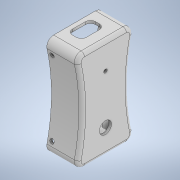
# Autodesk Inventor part: Bottom
Saved by Autodesk Inventor 2021 (Build 250183000, 183)
## iProperties
Created: 2024-02-01
Part Number: Bottom
Material: Generic
Document SubType Name: Modeling
Designer: maxsm
Density: 1 g/cm^3
Appearance: Default
Author: maxsm
Autodesk Inventor part; units mm, degrees
ref_plane "YZ Plane" through (0, 0, 0) normal (1, 0, 0) x (0, 1, 0)
ref_plane "XZ Plane" through (0, 0, 0) normal (0, 1, 0) x (-1, 0, 0)
ref_plane "XY Plane" through (0, 0, 0) normal (0, 0, 1) x (1, 0, 0)
sketch "Sketch1" plane through (0, 0, 0) normal (0, 1, 0) x (-1, 0, 0)
  line L0 (9, 13.5) -> (-9, 13.5)
  line L1 (-9, 13.5) -> (-9, -13.5)
  line L2 (-9, -13.5) -> (9, -13.5)
  line L3 (9, -13.5) -> (9, 13.5)
  line L4 (9, 13.5) -> (-9, -13.5) construction
  line L5 (-9, 13.5) -> (9, -13.5) construction
  point P0 (0, 0)
  dimension "d0" = 18
  dimension "d1" = 27
  constraints: 12 end point, 2 midpoint, 2 parallel, 1 horizontal, 1 perpendicular
  measures "d0" distance of L2.end L1.end
  measures "d1" distance of L1.end L0.end
extrude "Extrusion1" add sketch "Sketch1" along normal blind 58
sketch "Sketch5" plane through (-9, 0, -13.5) normal (-1, 0, 0) x (0, 0, 1)
  arc A0 (30.8, 58) -> (30.8, 0) centre (139.5579, 29) ccw
  line L0 (27, 58) -> (0, 58) projected
  line L1 (27, 58) -> (30.8, 58)
  line L2 (27, 0) -> (0, 0) projected
  line L3 (27, 0) -> (30.8, 0)
  line L4 (27, 0) -> (27, 58) projected
  arc A1 (-3.8, 0) -> (-3.8, 58) centre (-112.5579, 29) ccw
  line L5 (0, 58) -> (-3.8, 58)
  line L6 (0, 0) -> (-3.8, 0)
  line L7 (0, 0) -> (0, 58) projected
  point P0 (13.5, 0)
  point P1 (27, 29)
  point P2 (0, 29)
  dimension "d26" = 3.8
  constraints: 8 end point, 4 point on circle, 3 equal length, 3 horizontal, 2 centre point, 2 tangent, 1 collinear
  measures "d26" distance from line of L4 L1.end
extrude "Extrusion5" add sketch "Sketch5" against normal up to surface (18 mm away) contours A0 L4 L1 | A0 L3 L4 | L7 A1 L5 | L6 A1 L7
fillet "Fillet1" radius 2 4 edges at (9, 0, 0) (9, 58, 0) (9, 29, 13.5) (9, 29, -13.5)
fillet "Fillet1" radius 4 4 edges at (0, 58, -17.3) (0, 58, 17.3) (0, 0, 17.3) (0, 0, -17.3)
shell "Shell1" thickness 1.5 removed faces 1 at (-9, 11.2387, -4.0709)
sketch "Sketch6" plane through (7.5, 29, 126.0579) normal (-1, 0, 0) x (0, 0, 1)
  circle A0 centre (-117.1679, -21.22) radius 1.2
  circle A1 centre (-117.1679, -21.22) radius 2.5
  circle A2 centre (-134.9479, -21.22) radius 1.2
  circle A3 centre (-134.9479, -21.22) radius 2.5
  circle A4 centre (-117.1679, 24.5) radius 1.2
  circle A5 centre (-117.1679, 24.5) radius 2.5
  circle A6 centre (-134.9479, 24.5) radius 1.2
  circle A7 centre (-134.9479, 24.5) radius 2.5
  line L0 (-113.8453, -27.5) -> (-138.2705, -27.5) projected
  line L1 (-126.0579, -40.6) -> (-126.0579, 40.6) projected
  line L2 (-138.2705, 27.5) -> (-113.8453, 27.5) projected
  point P0 (-126.0579, -29)
  dimension "d33" = 5
  dimension "d34" = 2.4
  dimension "d36" = 17.78
  dimension "d37" = 45.72
  dimension "d40" = 3
  constraints: 8 centre point, 5 equal radius, 4 coincident, 2 horizontal alignment, 2 vertical alignment, 1 other
  measures "d33" diameter of A1
  measures "d34" diameter of A0
  measures "d36" distance of A2.centre A0.centre
  measures "d37" distance of A4.centre A0.centre
  measures "d40" distance from line of A4.centre L2
extrude "Extrusion6" add sketch "Sketch6" along normal blind 6.8
sketch "Sketch7" plane through (0, 58, 0) normal (0, 1, 0) x (1, 0, 0)
  line L0 (-2.4, -2.65) -> (-2.4, 2.65) construction
  line L1 (1.7, -2.65) -> (1.7, 2.65)
  line L2 (-6.5, 2.65) -> (-6.5, -2.65)
  arc A0 (-6.5, -2.65) -> (1.7, -2.65) centre (-2.4, -2.65) ccw
  arc A1 (1.7, 2.65) -> (-6.5, 2.65) centre (-2.4, 2.65) ccw
  line L3 (9, -12.2126) -> (9, 12.2126) projected
  line L4 (-6.5, -6.75) -> (1.7, -6.75)
  line L5 (1.7, -6.75) -> (1.7, 6.75)
  line L6 (1.7, 6.75) -> (-6.5, 6.75)
  line L7 (-6.5, 6.75) -> (-6.5, -6.75)
  point P0 (0, 0)
  point P1 (-2.4, 0)
  point P2 (-2.4, 6.75)
  point P3 (-2.4, -6.75)
  dimension "d41" = 11.4
  dimension "d42" = 8.2
  dimension "d43" = 13.5
  constraints: 16 end point, 6 point on circle, 4 tangent, 3 midpoint, 3 parallel, 2 centre point, 2 point on line, 1 horizontal, 1 horizontal alignment, 1 perpendicular, 1 vertical
  measures "d41" distance between parallel lines of L3 L0
  measures "d42" distance between parallel lines of L1 L2
extrude "Extrusion7" cut sketch "Sketch7" against normal blind 1.5
fillet "Fillet3" radius 3 4 edges at (1.7, 57.25, 6.75) (-6.5, 57.25, 6.75) (-6.5, 57.25, -6.75) (1.7, 57.25, -6.75)
sketch "Sketch8" plane through (7.5, 29, 126.0579) normal (-1, 0, 0) x (0, 0, 1)
  circle A0 centre (-134.9479, -21.22) radius 1.2 projected
  circle A1 centre (-134.9479, -21.22) radius 2.5 projected
  circle A2 centre (-117.1679, -21.22) radius 1.2 projected
  circle A3 centre (-117.1679, -21.22) radius 2.5 projected
  circle A4 centre (-134.9479, 24.5) radius 1.2 projected
  circle A5 centre (-117.1679, 24.5) radius 1.2 projected
  arc A6 (-113.8453, -27) -> (-111.8918, -24.571) centre (-113.8453, -25) ccw projected
  arc A7 (-111.8918, 24.571) -> (-111.8918, -24.571) centre (0, 0) ccw projected
  arc A8 (-111.8918, 24.571) -> (-113.8453, 27) centre (-113.8453, 25) ccw projected
  line L0 (-117.1679, 27) -> (-113.8453, 27) projected
  circle A9 centre (-117.1679, 24.5) radius 2.5 projected
  line L1 (-134.9479, 27) -> (-117.1679, 27) projected
  circle A10 centre (-134.9479, 24.5) radius 2.5 projected
  line L2 (-138.2705, 27) -> (-134.9479, 27) projected
  arc A11 (-138.2705, 27) -> (-140.224, 24.571) centre (-138.2705, 25) ccw projected
  arc A12 (-140.224, -24.571) -> (-140.224, 24.571) centre (-252.1158, 0) ccw projected
  arc A13 (-140.224, -24.571) -> (-138.2705, -27) centre (-138.2705, -25) ccw projected
  line L3 (-138.2705, -27) -> (-113.8453, -27) projected
  arc A14 (-113.8453, -28.9365) -> (-110.0004, -24.1557) centre (-113.8453, -25) ccw projected
  line L4 (-113.8453, -28.9365) -> (-138.2705, -28.9365) projected
  arc A15 (-142.1154, -24.1557) -> (-138.2705, -28.9365) centre (-138.2705, -25) ccw projected
  arc A16 (-142.1154, -24.1557) -> (-142.1154, 24.1557) centre (-252.1158, 0) ccw projected
  arc A17 (-138.2705, 28.9365) -> (-142.1154, 24.1557) centre (-138.2705, 25) ccw projected
  line L5 (-138.2705, 28.9365) -> (-113.8453, 28.9365) projected
  arc A18 (-110.0004, 24.1557) -> (-113.8453, 28.9365) centre (-113.8453, 25) ccw projected
  arc A19 (-110.0004, 24.1557) -> (-110.0004, -24.1557) centre (0, 0) ccw projected
  circle A20 centre (-126.0579, -14.87) radius 3.55
  line L6 (-126.0579, -41.8004) -> (-126.0579, 41.8004) projected
  circle A21 centre (-126.0579, 13.705) radius 1
  point P0 (-126.0579, -29)
  dimension "d47" = 39.37
  dimension "d48" = 7.1
  dimension "d49" = 2
  dimension "d50" = 10.795
  constraints: 2 centre point, 2 point on line, 2 vertical alignment
  measures "d47" vertical distance of A20.centre A5.centre
  measures "d48" diameter of A20
  measures "d49" diameter of A21
  measures "d50" vertical distance of A21.centre A5.centre
extrude "Extrusion8" cut sketch "Sketch8" against normal through all contours L6 A20 | A20 L6 | A21 L6 | L6 A21
sketch "Sketch13" plane through (-9, 29, 126.0579) normal (-1, 0, 0) x (0, 0, 1)
  arc A0 (-138.2705, 27.5) -> (-140.7123, 24.4638) centre (-138.2705, 25) ccw projected
  arc A1 (-140.7123, -24.4638) -> (-140.7123, 24.4638) centre (-252.1158, 0) ccw projected
  arc A2 (-140.7123, -24.4638) -> (-138.2705, -27.5) centre (-138.2705, -25) ccw projected
  line L0 (-138.2705, -27.5) -> (-113.8453, -27.5) projected
  arc A3 (-113.8453, -27.5) -> (-111.4034, -24.4638) centre (-113.8453, -25) ccw projected
  arc A4 (-111.4034, 24.4638) -> (-111.4034, -24.4638) centre (0, 0) ccw projected
  arc A5 (-111.4034, 24.4638) -> (-113.8453, 27.5) centre (-113.8453, 25) ccw projected
  line L1 (-113.8453, 27.5) -> (-138.2705, 27.5) projected
  arc A6 (-138.2705, 29) -> (-142.1774, 24.1421) centre (-138.2705, 25) ccw projected
  line L2 (-138.2705, 29) -> (-113.8453, 29) projected
  arc A7 (-109.9383, 24.1421) -> (-113.8453, 29) centre (-113.8453, 25) ccw projected
  arc A8 (-109.9383, 24.1421) -> (-109.9383, -24.1421) centre (0, 0) ccw projected
  arc A9 (-113.8453, -29) -> (-109.9383, -24.1421) centre (-113.8453, -25) ccw projected
  line L3 (-113.8453, -29) -> (-138.2705, -29) projected
  arc A10 (-142.1774, -24.1421) -> (-138.2705, -29) centre (-138.2705, -25) ccw projected
  arc A11 (-142.1774, -24.1421) -> (-142.1774, 24.1421) centre (-252.1158, 0) ccw projected
  arc A12 (-140.7123, -24.4638) -> (-140.7123, 24.4638) centre (-252.1158, 0) ccw projected
  point P0 (-126.0579, -29)
  point P1 (-139.7472, 19.5578)
  dimension "d74" = 5
  constraints: 1 point on circle
  measures "d74" distance of point (-139.747, 19.558) A0.end
ref_plane "Work Plane1" through (-9, 53.4638, -14.6545) normal (0, 0.1930256, 0.9811937) x (-1, 0, 0)
sketch "Sketch14" plane through (-9, 53.4638, -14.6545) normal (0, 0.1930256, 0.9811937) x (-1, 0, 0)
  circle A0 centre (-2.5, 2.5) radius 1.25
  line L0 (-21.6, 5) -> (3.6, 5) projected
  line L1 (0, 0) -> (0, 48.0074) projected
  point P0 (-9, 55.287)
  dimension "d75" = 2.5
  dimension "d76" = 2.5
  dimension "d77" = 2.5
  constraints: 1 centre point
  measures "d75" diameter of A0
  measures "d76" distance from line of L0 A0.centre
  measures "d77" distance from line of A0.centre L1
extrude "Extrusion13" cut sketch "Sketch14" against normal mid plane 10
mirror "Mirror3" about plane through (0, 0, 0) normal (0, 0, 1) of "Extrusion13"
ref_plane "Work Plane2" through (-9, 29, 12.2126) normal (0, -1, 0) x (1, 0, 0)
mirror "Mirror4" about plane through (-9, 29, 12.2126) normal (0, -1, 0) of "Extrusion13", "Mirror3"
sketch "Sketch15" plane through (-9, 53.4638, -14.6545) normal (0, 0.1930256, 0.9811937) x (-1, 0, 0)
  point P0 (-9, 55.287)
body "Solid1"
